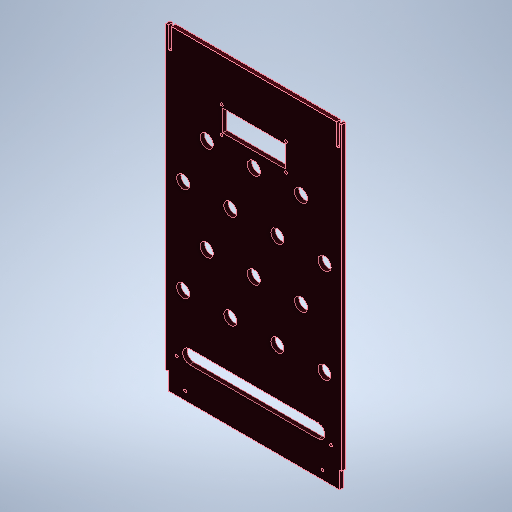
# Autodesk Inventor part: Random Plate  ( Laser Cut )
Saved by Autodesk Inventor 2025.4 (Build 294407000, 407)
## iProperties
Created: 2026-03-12
Part Number: Random Plate  ( Laser Cut )
Material: Generic
Document SubType Name: Sheet Metal
Designer: lenovo
Density: 1 g/cm^3
Sheet Metal Rule: Default_mm
Appearance: Default(3)
Author: lenovo
Autodesk Inventor part; units mm, degrees
ref_plane "YZ Plane" through (0, 0, 0) normal (1, 0, 0) x (0, 1, 0)
ref_plane "XZ Plane" through (0, 0, 0) normal (0, 1, 0) x (-1, 0, 0)
sketch "Sketch1" plane through (0, 0, 0) normal (0, 0, 1) x (1, 0, 0)
  line L0 (0, 0) -> (200, 0)
  line L1 (200, 0) -> (200, 370)
  line L2 (200, 370) -> (0, 370)
  line L3 (0, 370) -> (0, 0)
  circle A0 centre (17.5, 330) radius 7.6
  circle A1 centre (72.5, 330) radius 7.6
  circle A2 centre (127.5, 330) radius 7.6
  circle A3 centre (182.5, 330) radius 7.6
  circle A4 centre (45, 275) radius 7.6
  circle A5 centre (100, 275) radius 7.6
  circle A6 centre (155, 275) radius 7.6
  circle A7 centre (17.5, 220) radius 7.6
  circle A8 centre (72.5, 220) radius 7.6
  circle A9 centre (127.5, 220) radius 7.6
  circle A10 centre (182.5, 220) radius 7.6
  circle A11 centre (17.5, 110) radius 7.6
  circle A12 centre (72.5, 110) radius 7.6
  circle A13 centre (127.5, 110) radius 7.6
  circle A14 centre (182.5, 110) radius 7.6
  circle A15 centre (45, 165) radius 7.6
  circle A16 centre (100, 165) radius 7.6
  circle A17 centre (155, 165) radius 7.6
  line L4 (0, 370) -> (-2.5, 370)
  line L5 (-2.5, 370) -> (-2.5, 20)
  line L6 (-2.5, 20) -> (0, 20)
  line L7 (0, 20) -> (0, 370)
  line L8 (200, 370) -> (202.5, 370)
  line L9 (202.5, 370) -> (202.5, 20)
  line L10 (202.5, 20) -> (200, 20)
  line L11 (200, 20) -> (200, 370)
  point P0 (0, 20)
  dimension "d16" = 200
  dimension "d17" = 370
  dimension "d18" = 15.2
  dimension "d19" = 40
  dimension "d20" = 17.5
  dimension "d21" = 55
  dimension "d22" = 55
  dimension "d23" = 45
  dimension "d24" = 55
  dimension "d25" = 110
  dimension "d26" = 110
  dimension "d95" = 2.5
  dimension "d96" = 20
  dimension "d97" = 2.5
  dimension "d98" = 20
  measures "d16" distance between parallel lines of L1 L3
  measures "d17" distance between parallel lines of L0 L2
  measures "d18" diameter of A0
  measures "d19" distance from line of L2 A0.centre
  measures "d20" distance from line of L3 A0.centre
  measures "d21" distance of A0.centre A1.centre
  measures "d22" vertical distance of A0.centre A4.centre
  measures "d23" distance from line of L3 A4.centre
  measures "d24" distance of A4.centre A5.centre
  measures "d25" distance of A0.centre A7.centre
  measures "d26" distance of A4.centre A15.centre
  measures "d95" distance of L3.start L4.end
  measures "d96" distance between parallel lines of L0 L6
  measures "d97" distance of L9.end L10.end
  measures "d98" distance between parallel lines of L0 L10
extrude "Plate1" add sketch "Sketch1" along normal blind 5 contours L3 L2 L1 L0 | L6 L5 L4 L3 | L1 L8 L9 L10 | A0 | A1 | A2 | A3
sketch "Sketch2" plane through (0, 0, 5) normal (0, 0, 1) x (1, 0, 0)
  line L0 (25, 47) -> (175, 47) construction
  line L1 (25, 39) -> (175, 39)
  line L2 (175, 55) -> (25, 55)
  arc A0 (25, 55) -> (25, 39) centre (25, 47) ccw
  arc A1 (175, 39) -> (175, 55) centre (175, 47) ccw
  line L3 (0, 0) -> (0, 20) projected
  line L4 (200, 20) -> (200, 0) projected
  circle A2 centre (127.5, 110) radius 7.6 projected
  line L5 (200, 0) -> (0, 0) projected
  point P0 (100, 47)
  point P1 (0, 370)
  point P2 (200, 370)
  point P3 (100, 0)
  dimension "d32" = 16
  dimension "d35" = 55
  dimension "d39" = 150
  constraints: 8 end point, 4 point on circle, 4 tangent, 2 centre point, 2 midpoint, 1 horizontal, 1 parallel, 1 vertical alignment
  measures "d32" distance between parallel lines of L1 L2
  measures "d35" distance from line of L2 A2.centre
  measures "d39" distance of L0.end L0.start
extrude "Cut1" cut sketch "Sketch2" against normal through all contours A0 L2 A1 L1
sketch "Sketch3" plane through (0, 0, 5) normal (0, 0, 1) x (1, 0, 0)
  circle A0 centre (10, 40.1) radius 1.65
  line L0 (175, 39) -> (25, 39) projected
  line L1 (100, 39) -> (100, 0)
  line L2 (200, 0) -> (0, 0) projected
  circle A1 centre (190, 40.1) radius 1.65
  dimension "d41" = 3.3
  dimension "d47" = 180
  dimension "d48" = 1.1
  constraints: 3 midpoint, 2 centre point, 2 end point, 1 perpendicular, 1 symmetric about line, 1 vertical alignment, 1 other
  measures "d41" diameter of A0
  measures "d47" diameter of A0.centre L1
  measures "d48" distance from line of A0.centre L0
extrude "Cut2" cut sketch "Sketch3" against normal blind 5
sketch "Sketch4" plane through (0, 0, 5) normal (0, 0, 1) x (1, 0, 0)
  line L0 (60, 322.5) -> (140, 322.5)
  line L1 (140, 322.5) -> (140, 287.5)
  line L2 (140, 287.5) -> (60, 287.5)
  line L3 (60, 287.5) -> (60, 322.5)
  line L4 (60, 322.5) -> (140, 287.5) construction
  line L5 (140, 322.5) -> (60, 287.5) construction
  line L6 (63.5, 317.5) -> (136.5, 317.5)
  line L7 (136.5, 317.5) -> (136.5, 292.5)
  line L8 (136.5, 292.5) -> (63.5, 292.5)
  line L9 (63.5, 292.5) -> (63.5, 317.5)
  line L10 (63.5, 317.5) -> (136.5, 292.5) construction
  line L11 (136.5, 317.5) -> (63.5, 292.5) construction
  line L12 (-2.5, 370) -> (202.5, 370) projected
  circle A0 centre (100, 275) radius 7.6 projected
  circle A1 centre (137.5, 320.5) radius 1.65
  line L13 (100, 317.5) -> (100, 292.5)
  line L14 (63.5, 305) -> (136.5, 305)
  circle A2 centre (62.5, 320.5) radius 1.65
  circle A3 centre (137.5, 289.5) radius 1.65
  circle A4 centre (62.5, 289.5) radius 1.65
  point P0 (0, 0)
  point P1 (100, 305)
  point P2 (100, 305)
  point P3 (100, 370)
  point P4 (5, 370)
  point P5 (195, 370)
  point P6 (100, 305)
  dimension "d50" = 30
  dimension "d51" = 35
  dimension "d52" = 80
  dimension "d53" = 73
  dimension "d54" = 25
  dimension "d55" = 3.3
  dimension "d101" = 31
  dimension "d102" = 75
  constraints: 28 end point, 10 midpoint, 4 centre point, 4 parallel, 3 symmetric about line, 2 horizontal, 2 perpendicular, 1 vertical alignment, 3 other
  measures "d50" distance of A0.centre point (100, 305)
  measures "d51" distance of L2.end L0.start
  measures "d52" distance of L0.start L0.end
  measures "d53" distance of L6.start L6.end
  measures "d54" distance of L8.end L6.start
  measures "d55" diameter of A1
  measures "d101" diameter of A1.centre L14
  measures "d102" diameter of A1.centre L13
extrude "Extrusion1" cut sketch "Sketch4" against normal blind 10 contours L6 L13 L14 L9 | L6 L7 L14 L13 | L14 L13 L8 L9 | L14 L7 L8 L13 | A1 | A2 | A3 | A4
sketch "Sketch8" plane through (0, 0, 5) normal (0, 0, 1) x (1, 0, 0)
  line L0 (202.5, 370) -> (-2.5, 370) projected
  line L1 (196.5, 370) -> (199.5, 370)
  line L2 (199.5, 370) -> (199.5, 345)
  line L3 (199.5, 345) -> (196.5, 345)
  line L4 (196.5, 345) -> (196.5, 370)
  line L5 (200, 20) -> (200, 0) projected
  line L6 (202.5, 370) -> (202.5, 20) projected
  point P0 (0, 0)
  point P1 (195, 370)
  point P2 (5, 370)
  point P3 (200, 365)
  dimension "d76" = 25
  dimension "d77" = 3
  dimension "d99" = 3
  constraints: 8 end point, 2 parallel, 1 horizontal, 1 perpendicular, 1 point on line
  measures "d76" distance of L1.end L2.end
  measures "d77" distance of L2.end L3.end
  measures "d99" distance between parallel lines of L6 L2
extrude "Cut6" cut sketch "Sketch8" against normal blind 5
sketch "Sketch9" plane through (0, 0, 5) normal (0, 0, 1) x (1, 0, 0)
  line L0 (196.5, 370) -> (199.5, 370) projected
  line L1 (3.5, 370) -> (0.5, 370)
  line L2 (0.5, 370) -> (0.5, 345)
  line L3 (0.5, 345) -> (3.5, 345)
  line L4 (3.5, 345) -> (3.5, 370)
  line L5 (0, 0) -> (0, 20) projected
  line L6 (-2.5, 20) -> (-2.5, 370) projected
  point P0 (5, 370)
  point P1 (0, 365)
  point P2 (5, 370)
  dimension "d81" = 25
  dimension "d82" = 3
  dimension "d100" = 3
  constraints: 8 end point, 2 parallel, 1 horizontal, 1 perpendicular, 1 point on line
  measures "d81" distance of L3.end L1.start
  measures "d82" distance of L2.end L3.end
  measures "d100" distance between parallel lines of L6 L2
extrude "Cut7" cut sketch "Sketch9" against normal blind 5
sketch "Sketch10" plane through (0, 0, 5) normal (0, 0, 1) x (1, 0, 0)
  circle A0 centre (180, 10) radius 1.65
  line L0 (200, 20) -> (200, 0) projected
  line L1 (200, 0) -> (0, 0) projected
  circle A1 centre (20, 10) radius 1.65
  line L2 (0, 0) -> (0, 20) projected
  point P0 (200, 365)
  point P1 (0, 365)
  dimension "d86" = 3.3
  dimension "d88" = 10
  dimension "d89" = 3.3
  dimension "d90" = 10
  dimension "d91" = 20
  dimension "d94" = 20
  constraints: 2 centre point
  measures "d86" diameter of A0
  measures "d88" distance from line of L1 A0.centre
  measures "d89" diameter of A1
  measures "d90" distance from line of L1 A1.centre
  measures "d91" distance from line of L2 A1.centre
  measures "d94" distance from line of L0 A0.centre
extrude "Cut8" cut sketch "Sketch10" against normal blind 5
ref_plane "Work Plane1" through (100, 20, 0) normal (1, 0, 0) x (0, 0, -1)
equation "\"d97\" = d95"
equation "\"d98\" = d96"
equation "\"d36\" = Thickness"
equation "\"d45\" = Thickness"
equation "\"d79\" = Thickness"
equation "\"d84\" = Thickness"
equation "\"d92\" = Thickness"
equation "\"d31\" = Thickness"
equation "\"BendRadius\" = Thickness"
equation "\"BendReliefWidth\" = Thickness"
equation "\"BendReliefDepth\" = 0.5 * Thickness"
equation "\"TransitionRadius\" = BendRadius"
equation "\"JacobiRadiusSize\" = BendRadius"
equation "\"GapSize\" = Thickness"
equation "\"Thickness\" = 5"
body "Solid1"
